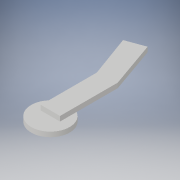
# Autodesk Inventor part: scale_r_arm
Saved by Autodesk Inventor 2018 (Build 220112000, 112)
## iProperties
Created: 2018-05-04
Part Number: scale_r_arm
Material: Generic
Document SubType Name: Modeling
Designer: 4070609
Density: 1 g/cm^3
Appearance: Default
Author: 4070609
Autodesk Inventor part; units mm, degrees
ref_plane "YZ Plane" through (0, 0, 0) normal (1, 0, 0) x (0, 1, 0)
ref_plane "XZ Plane" through (0, 0, 0) normal (0, 1, 0) x (-1, 0, 0)
ref_plane "XY Plane" through (0, 0, 0) normal (0, 0, 1) x (1, 0, 0)
sketch "Sketch1" plane through (0, 0, 0) normal (0, 1, 0) x (-1, 0, 0)
  circle A0 centre (0, 0) radius 20
  dimension "d0" = 40
  constraints: 1 centre point, 1 coincident
  measures "d0" diameter of A0
extrude "Extrusion1" add sketch "Sketch1" along normal blind 5
sketch "Sketch2" plane through (0, 5, 0) normal (0, 1, 0) x (1, 0, 0)
  line L0 (0, 0) -> (-10, 0)
  line L1 (-10, 0) -> (-10, 60)
  line L2 (-10, 60) -> (0, 60)
  line L3 (0, 60) -> (0, 0)
  line L4 (0, 0) -> (10, 0)
  line L5 (10, 0) -> (10, 60)
  line L6 (10, 60) -> (0, 60)
  line L7 (0, 60) -> (0, 0)
  line L8 (0, 60) -> (-16.246, 104.6354)
  line L9 (0, 60) -> (-9.3969, 56.5798)
  line L10 (-9.3969, 56.5798) -> (-25.6429, 101.2152)
  line L11 (-25.6429, 101.2152) -> (-16.246, 104.6354)
  line L12 (-16.246, 104.6354) -> (-6.849, 108.0556)
  line L13 (-6.849, 108.0556) -> (10, 60)
  dimension "d3" = 10
  dimension "d4" = 60
  dimension "d5" = 10
  dimension "d7" = 47.5
  dimension "d8" = 160
  dimension "d9" = 10
  dimension "d10" = 10
  constraints: 28 end point, 4 parallel, 4 perpendicular, 2 horizontal, 1 point on line
  measures "d3" distance of L1.end L2.end
  measures "d4" distance of L0.end L1.end
  measures "d5" distance of L6.end L5.end
  measures "d7" distance of L6.end L8.end
  measures "d8" angle of L8 L3
  measures "d9" distance of L6.end L9.end
  measures "d10" distance of L8.end L12.end
extrude "Extrusion2" add sketch "Sketch2" along normal blind 5
body "Solid1"
